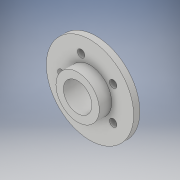
# Autodesk Inventor part: PVC motor gear
Saved by Autodesk Inventor 2017 (Build 210142000, 142)
## iProperties
Created: 2017-05-04
Part Number: PVC motor gear
Material: Generic
Document SubType Name: Modeling
Designer: Jon
Density: 1 g/cm^3
Appearance: Default
Author: Jon
Autodesk Inventor part; units mm, degrees
ref_plane "YZ Plane" through (0, 0, 0) normal (1, 0, 0) x (0, 1, 0)
ref_plane "XZ Plane" through (0, 0, 0) normal (0, 1, 0) x (-1, 0, 0)
ref_plane "XY Plane" through (0, 0, 0) normal (0, 0, 1) x (1, 0, 0)
sketch "Sketch1" plane through (0, 0, 0) normal (0, 0, 1) x (1, 0, 0)
  line L0 (-25.1788, 61.8531) -> (-25.1788, 68.2031)
  line L1 (-13.5921, 60.3277) -> (-11.9486, 66.4613)
  line L2 (-2.7951, 55.8554) -> (0.3799, 61.3547)
  line L3 (6.4766, 48.741) -> (10.9667, 53.2312)
  line L4 (13.591, 39.4694) -> (19.0902, 42.6444)
  line L5 (18.0633, 28.6723) -> (24.1969, 30.3158)
  line L6 (19.5887, 17.0856) -> (25.9387, 17.0856)
  line L7 (18.0633, 5.4989) -> (24.1969, 3.8554)
  line L8 (13.591, -5.2981) -> (19.0902, -8.4731)
  line L9 (6.4766, -14.5698) -> (10.9667, -19.0599)
  line L10 (-2.7951, -21.6842) -> (0.3799, -27.1834)
  line L11 (-13.5921, -26.1565) -> (-11.9486, -32.2901)
  line L12 (-25.1788, -27.6819) -> (-25.1788, -34.0319)
  line L13 (-36.7655, -26.1565) -> (-38.409, -32.2901)
  line L14 (-47.5626, -21.6842) -> (-50.7376, -27.1834)
  line L15 (-56.8342, -14.5698) -> (-61.3243, -19.0599)
  line L16 (-63.9486, -5.2981) -> (-69.4479, -8.4731)
  line L17 (-68.4209, 5.4989) -> (-74.5545, 3.8554)
  line L18 (-69.9463, 17.0856) -> (-76.2963, 17.0856)
  line L19 (-68.4209, 28.6723) -> (-74.5545, 30.3158)
  line L20 (-63.9486, 39.4694) -> (-69.4479, 42.6444)
  line L21 (-56.8342, 48.741) -> (-61.3243, 53.2312)
  line L22 (-47.5626, 55.8554) -> (-50.7376, 61.3547)
  line L23 (-36.7655, 60.3277) -> (-38.409, 66.4613)
  arc A0 (-38.409, 66.4613) -> (-25.1788, 68.2031) centre (-31.8994, 68.1336) ccw
  arc A1 (-25.1788, 68.2031) -> (-11.9486, 66.4613) centre (-18.4582, 68.1336) ccw
  arc A2 (-11.9486, 66.4613) -> (0.3799, 61.3547) centre (-5.475, 64.6547) ccw
  arc A3 (0.3799, 61.3547) -> (10.9667, 53.2312) centre (6.1654, 57.9342) ccw
  arc A4 (10.9667, 53.2312) -> (19.0902, 42.6444) centre (15.6697, 48.4298) ccw
  arc A5 (19.0902, 42.6444) -> (24.1969, 30.3158) centre (22.3903, 36.7894) ccw
  arc A6 (24.1969, 30.3158) -> (25.9387, 17.0856) centre (25.8692, 23.8062) ccw
  arc A7 (25.9387, 17.0856) -> (24.1969, 3.8554) centre (25.8692, 10.365) ccw
  arc A8 (24.1969, 3.8554) -> (19.0902, -8.4731) centre (22.3903, -2.6182) ccw
  arc A9 (19.0902, -8.4731) -> (10.9667, -19.0599) centre (15.6697, -14.2586) ccw
  arc A10 (10.9667, -19.0599) -> (0.3799, -27.1834) centre (6.1654, -23.7629) ccw
  arc A11 (0.3799, -27.1834) -> (-11.9486, -32.2901) centre (-5.475, -30.4835) ccw
  arc A12 (-11.9486, -32.2901) -> (-25.1788, -34.0319) centre (-18.4582, -33.9623) ccw
  arc A13 (-25.1788, -34.0319) -> (-38.409, -32.2901) centre (-31.8994, -33.9623) ccw
  arc A14 (-38.409, -32.2901) -> (-50.7376, -27.1834) centre (-44.8826, -30.4835) ccw
  arc A15 (-50.7376, -27.1834) -> (-61.3243, -19.0599) centre (-56.523, -23.7629) ccw
  arc A16 (-61.3243, -19.0599) -> (-69.4479, -8.4731) centre (-66.0273, -14.2586) ccw
  arc A17 (-69.4479, -8.4731) -> (-74.5545, 3.8554) centre (-72.7479, -2.6182) ccw
  arc A18 (-74.5545, 3.8554) -> (-76.2963, 17.0856) centre (-76.2268, 10.365) ccw
  arc A19 (-76.2963, 17.0856) -> (-74.5545, 30.3158) centre (-76.2268, 23.8062) ccw
  arc A20 (-74.5545, 30.3158) -> (-69.4479, 42.6444) centre (-72.7479, 36.7894) ccw
  arc A21 (-69.4479, 42.6444) -> (-61.3243, 53.2312) centre (-66.0273, 48.4298) ccw
  arc A22 (-61.3243, 53.2312) -> (-50.7376, 61.3547) centre (-56.523, 57.9342) ccw
  arc A23 (-50.7376, 61.3547) -> (-38.409, 66.4613) centre (-44.8826, 64.6547) ccw
  circle A24 centre (-25.1788, 17.0856) radius 44.7675
  point P0 (0, 0)
  dimension "d36" = 89.535
  dimension "d8" = 360
  constraints: 48 end point, 48 point on circle, 24 centre point, 3 coincident, 1 horizontal alignment, 1 vertical, 193 other
extrude "Extrusion1" add sketch "Sketch1" along normal blind 6.35 contours A24
sketch "Sketch2" plane through (-25.1788, 17.0856, 0) normal (0, 0, -1) x (-1, 0, 0)
  circle A0 centre (-23.7729, 17.272) radius 3.81
  circle A1 centre (0, 0) radius 44.7675 projected
  circle A2 centre (9.0804, 27.9467) radius 3.81
  circle A3 centre (29.3849, 0) radius 3.81
  circle A4 centre (9.0804, -27.9467) radius 3.81
  circle A5 centre (-23.7729, -17.272) radius 3.81
  point P0 (-25.1788, -17.0856)
  dimension "d15" = 360
  dimension "d17" = 17.272
  dimension "d19" = 0
  dimension "d20" = 7.62
  constraints: 5 centre point, 2 coincident, 13 other
  measures "d17" vertical distance of A0.centre A1.centre
  measures "d19" vertical distance of A3.centre A1.centre
  measures "d20" diameter of A0
hole "Hole1" at (-1.4059, 34.3576, 0) at (-1.4059, -0.1864, 0) at (-34.2592, 45.0323, 0) at (-34.2592, -10.8611, 0) at (-54.5637, 17.0856, 0) direction (0, 0, 1) diameter 7.62 end through all
sketch "Sketch3" plane through (-25.1788, 17.0856, 0) normal (0, 0, -1) x (-1, 0, 0)
  point P0 (-25.1788, -17.0856)
sketch "Sketch4" plane through (-25.1788, 17.0856, 0) normal (0, 0, -1) x (-1, 0, 0)
  point P0 (-25.1788, -17.0856)
sketch "Sketch6" plane through (-25.1788, 17.0856, 6.35) normal (0, 0, 1) x (1, 0, 0)
  circle A0 centre (0, 0) radius 14.605
  point P0 (25.1788, -17.0856)
  dimension "d48" = 29.21
  constraints: 1 centre point
  measures "d48" diameter of A0
sketch "Sketch7" plane through (-25.1788, 17.0856, 6.35) normal (0, 0, 1) x (1, 0, 0)
  circle A0 centre (0, 0) radius 22.225
  point P0 (25.1788, -17.0856)
  dimension "d51" = 44.45
  constraints: 1 centre point
  measures "d51" diameter of A0
extrude "Extrusion4" add sketch "Sketch7" along normal mid plane 25.4
extrude "Extrusion5" cut sketch "Sketch6" along normal through all both and the other way through all
body "Solid1"
